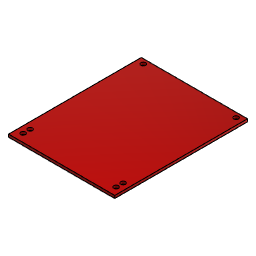
4ちゃん (Autodesk Fusion 360 design; units mm, degrees)
Autodesk Fusion 360 part; units mm, degrees
note: some values were not read from the file. Set by a fixed rule: which sketch regions a step uses.
sketch "スケッチ1" plane through (0, 0, 0) normal (0, 1, 0) x (1, 0, 0)
  line L0 (-40, -50) -> (40, -50)
  line L1 (40, -50) -> (40, 50)
  line L2 (40, 50) -> (-40, 50)
  line L3 (-40, 50) -> (-40, -50)
  line L4 (-40, -50) -> (40, 50) construction
  line L5 (40, -50) -> (-40, 50) construction
  dimension "d1" = 80
  dimension "d2" = 100
  constraint perpendicular L0 L1
  constraint parallel L0 L2
  constraint parallel L1 L3
  constraint horizontal L0
  constraint coincident L4 origin
  constraint coincident L5 origin
  measures "d1" distance of L1.end L2.end
  measures "d2" distance of L0.end L1.end
extrude "押し出し1" add sketch "スケッチ1" along normal blind 2
sketch "スケッチ2" plane through (0, 2, 0) normal (0, 1, 0) x (-1, 0, 0)
  line L0 (40, -50) -> (40, 50)
  line L1 (40, 50) -> (-40, 50)
  line L2 (-40, 50) -> (-40, -50)
  line L3 (-40, -50) -> (40, -50)
  line L4 (0, -50) -> (0, -46.5)
  line L5 (0, -46.5) -> (35, -46.5)
  line L6 (0, -46.5) -> (-35, -46.5)
  circle A0 centre (35, -46.5) radius 1.75
  circle A1 centre (-35, -46.5) radius 1.75
  line L7 (35, -46.5) -> (35, 44)
  circle A2 centre (35, 44) radius 1.75
  line L8 (35, 44) -> (-35, 44)
  circle A3 centre (-35, 44) radius 1.75
  dimension "d5" = 3.5
  dimension "d6" = 35
  dimension "d7" = 35
  dimension "d8" = 3.5
  dimension "d9" = 3.5
  dimension "d10" = 90.5
  dimension "d11" = 3.5
  dimension "d12" = 70
  dimension "d13" = 3.5
  constraint midpoint L3 L4.start
  constraint perpendicular L3 L4
  constraint perpendicular L4 L5
  constraint perpendicular L4 L6
  constraint coincident L5.end A0.centre
  constraint coincident L6.end A1.centre
  constraint perpendicular L5 L7
  constraint coincident L7.end A2.centre
  constraint perpendicular L7 L8
  constraint coincident L8.end A3.centre
  measures "d5" distance of L4.start L4.end
  measures "d6" distance of L4.end L5.end
  measures "d7" distance of L4.end L6.end
  measures "d8" diameter of A0
  measures "d9" diameter of A1
  measures "d10" distance of L5.end L7.end
  measures "d11" diameter of A2
  measures "d12" distance of L7.end L8.end
  measures "d13" diameter of A3
extrude "押し出し2" cut sketch "スケッチ2" against normal blind 5 contours L5 A0 L7 | L5 A0 L7 | A1 | L7 A2 L8 | L7 A2 L8 | A3
sketch "スケッチ3" plane through (0, 2, 0) normal (0, 1, 0) x (-1, 0, 0)
  circle A0 centre (35, -46.5) radius 1.75
  circle A1 centre (35, 44) radius 1.75
  circle A2 centre (-35, -46.5) radius 1.75
  circle A3 centre (-35, 44) radius 1.75
  line L0 (40, -50) -> (40, 50)
  line L1 (40, 50) -> (-40, 50)
  line L2 (-40, 50) -> (-40, -50)
  line L3 (-40, -50) -> (40, -50)
  line L4 (35, 44) -> (35, 38.71)
  line L5 (-35, 44) -> (-35, 38.71)
  circle A4 centre (35, 38.71) radius 1.75
  circle A5 centre (-35, 38.71) radius 1.75
  dimension "d16" = 5.29
  dimension "d17" = 5.29
  dimension "d18" = 3.5
  dimension "d19" = 3.5
  constraint coincident A1.centre L4.start
  constraint perpendicular L1 L4
  constraint coincident A3.centre L5.start
  constraint parallel L2 L5
  constraint coincident L4.end A4.centre
  constraint coincident L5.end A5.centre
  measures "d16" distance of A1.centre L4.end
  measures "d17" distance of A3.centre L5.end
  measures "d18" diameter of A4
  measures "d19" diameter of A5
extrude "押し出し3" cut sketch "スケッチ3" against normal blind 14 contours A4 | A5
